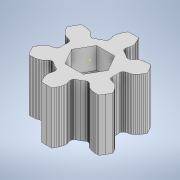
# Autodesk Inventor part: smallgears
Saved by Autodesk Inventor 2020 (Build 240168000, 168)
## iProperties
Created: 2019-08-05
Part Number: smallgears
Material: Generic
Document SubType Name: Modeling
Designer: erwin
Density: 1 g/cm^3
Appearance: Default
Author: erwin
Autodesk Inventor part; units mm, degrees
ref_plane "YZ Plane" through (0, 0, 0) normal (1, 0, 0) x (0, 1, 0)
ref_plane "XZ Plane" through (0, 0, 0) normal (0, 1, 0) x (-1, 0, 0)
ref_plane "XY Plane" through (0, 0, 0) normal (0, 0, 1) x (1, 0, 0)
sketch "Sketch1" plane through (0, 0, 0) normal (0, 1, 0) x (-1, 0, 0)
  line L0 (-11.846, 1.6672) -> (-11.8965, 2.1804)
  line L1 (-11.8965, 2.1804) -> (-11.9911, 2.3941)
  line L2 (-11.9911, 2.3941) -> (-12.094, 2.5558)
  line L3 (-12.094, 2.5558) -> (-12.2017, 2.6894)
  line L4 (-12.2017, 2.6894) -> (-12.3128, 2.8042)
  line L5 (-12.3128, 2.8042) -> (-12.4267, 2.905)
  line L6 (-12.4267, 2.905) -> (-12.6608, 3.0756)
  line L7 (-12.6608, 3.0756) -> (-12.902, 3.2145)
  line L8 (-12.902, 3.2145) -> (-13.1492, 3.3288)
  line L9 (-13.1492, 3.3288) -> (-13.6584, 3.4985)
  line L10 (-13.6584, 3.4985) -> (-14.1841, 3.6039)
  line L11 (-14.1841, 3.6039) -> (-14.7177, 3.6783)
  line L12 (-14.7177, 3.6783) -> (-15.2047, 3.9342)
  line L13 (-15.2047, 3.9342) -> (-15.6715, 4.2604)
  line L14 (-15.6715, 4.2604) -> (-16.1201, 4.6417)
  line L15 (-16.1201, 4.6417) -> (-16.5502, 5.0711)
  line L16 (-16.5502, 5.0711) -> (-16.961, 5.5447)
  line L17 (-16.961, 5.5447) -> (-17.3511, 6.0596)
  line L18 (-17.3511, 6.0596) -> (-17.7193, 6.6135)
  line L19 (-17.7193, 6.6135) -> (-18.064, 7.2045)
  line L20 (-18.064, 7.2045) -> (-18.3837, 7.831)
  line L21 (-18.3837, 7.831) -> (-17.3212, 9.9528)
  line L22 (-17.3212, 9.9528) -> (-16.0149, 11.9338)
  line L23 (-16.0149, 11.9338) -> (-15.3126, 11.9701)
  line L24 (-15.3126, 11.9701) -> (-14.6284, 11.9671)
  line L25 (-14.6284, 11.9671) -> (-13.9646, 11.9252)
  line L26 (-13.9646, 11.9252) -> (-13.3236, 11.8448)
  line L27 (-13.3236, 11.8448) -> (-12.7081, 11.7259)
  line L28 (-12.7081, 11.7259) -> (-12.1211, 11.5681)
  line L29 (-12.1211, 11.5681) -> (-11.5667, 11.3702)
  line L30 (-11.5667, 11.3702) -> (-11.0507, 11.1291)
  line L31 (-11.0507, 11.1291) -> (-10.5856, 10.8353)
  line L32 (-10.5856, 10.8353) -> (-10.2544, 10.4104)
  line L33 (-10.2544, 10.4104) -> (-9.9002, 10.0077)
  line L34 (-9.9002, 10.0077) -> (-9.4987, 9.6517)
  line L35 (-9.4987, 9.6517) -> (-9.2761, 9.4948)
  line L36 (-9.2761, 9.4948) -> (-9.0352, 9.3553)
  line L37 (-9.0352, 9.3553) -> (-8.7704, 9.2378)
  line L38 (-8.7704, 9.2378) -> (-8.6261, 9.1897)
  line L39 (-8.6261, 9.1897) -> (-8.4712, 9.1509)
  line L40 (-8.4712, 9.1509) -> (-8.3017, 9.1244)
  line L41 (-8.3017, 9.1244) -> (-8.1102, 9.1161)
  line L42 (-8.1102, 9.1161) -> (-7.8778, 9.141)
  line L43 (-7.8778, 9.141) -> (-7.4081, 9.3539)
  line L44 (-7.4081, 9.3539) -> (-5.9851, 10.318)
  line L45 (-5.9851, 10.318) -> (-4.4386, 11.0683)
  line L46 (-4.4386, 11.0683) -> (-4.0194, 11.3686)
  line L47 (-4.0194, 11.3686) -> (-3.8816, 11.5575)
  line L48 (-3.8816, 11.5575) -> (-3.7931, 11.7274)
  line L49 (-3.7931, 11.7274) -> (-3.7313, 11.8875)
  line L50 (-3.7313, 11.8875) -> (-3.6874, 12.0411)
  line L51 (-3.6874, 12.0411) -> (-3.657, 12.1901)
  line L52 (-3.657, 12.1901) -> (-3.6263, 12.4781)
  line L53 (-3.6263, 12.4781) -> (-3.6266, 12.7565)
  line L54 (-3.6266, 12.7565) -> (-3.6512, 13.0277)
  line L55 (-3.6512, 13.0277) -> (-3.7588, 13.5535)
  line L56 (-3.7588, 13.5535) -> (-3.9304, 14.0615)
  line L57 (-3.9304, 14.0615) -> (-4.1328, 14.5608)
  line L58 (-4.1328, 14.5608) -> (-4.1547, 15.1105)
  line L59 (-4.1547, 15.1105) -> (-4.1055, 15.6779)
  line L60 (-4.1055, 15.6779) -> (-3.9997, 16.257)
  line L61 (-3.9997, 16.257) -> (-3.8428, 16.8442)
  line L62 (-3.8428, 16.8442) -> (-3.6381, 17.4367)
  line L63 (-3.6381, 17.4367) -> (-3.3872, 18.0321)
  line L64 (-3.3872, 18.0321) -> (-3.0916, 18.6279)
  line L65 (-3.0916, 18.6279) -> (-2.7521, 19.2219)
  line L66 (-2.7521, 19.2219) -> (-2.3695, 19.812)
  line L67 (-2.3695, 19.812) -> (-0.0007, 19.9528)
  line L68 (-0.0007, 19.9528) -> (2.3681, 19.812)
  line L69 (2.3681, 19.812) -> (2.7507, 19.2219)
  line L70 (2.7507, 19.2219) -> (3.0902, 18.6279)
  line L71 (3.0902, 18.6279) -> (3.3858, 18.0321)
  line L72 (3.3858, 18.0321) -> (3.6366, 17.4367)
  line L73 (3.6366, 17.4367) -> (3.8414, 16.8442)
  line L74 (3.8414, 16.8442) -> (3.9983, 16.257)
  line L75 (3.9983, 16.257) -> (4.1041, 15.6779)
  line L76 (4.1041, 15.6779) -> (4.1533, 15.1105)
  line L77 (4.1533, 15.1105) -> (4.1314, 14.5608)
  line L78 (4.1314, 14.5608) -> (3.929, 14.0615)
  line L79 (3.929, 14.0615) -> (3.7574, 13.5535)
  line L80 (3.7574, 13.5535) -> (3.6498, 13.0277)
  line L81 (3.6498, 13.0277) -> (3.6252, 12.7565)
  line L82 (3.6252, 12.7565) -> (3.6249, 12.4781)
  line L83 (3.6249, 12.4781) -> (3.6555, 12.1901)
  line L84 (3.6555, 12.1901) -> (3.686, 12.0411)
  line L85 (3.686, 12.0411) -> (3.7298, 11.8875)
  line L86 (3.7298, 11.8875) -> (3.7917, 11.7274)
  line L87 (3.7917, 11.7274) -> (3.8802, 11.5575)
  line L88 (3.8802, 11.5575) -> (4.018, 11.3686)
  line L89 (4.018, 11.3686) -> (4.4372, 11.0683)
  line L90 (4.4372, 11.0683) -> (5.9837, 10.318)
  line L91 (5.9837, 10.318) -> (7.4067, 9.3539)
  line L92 (7.4067, 9.3539) -> (7.8764, 9.141)
  line L93 (7.8764, 9.141) -> (8.1088, 9.1161)
  line L94 (8.1088, 9.1161) -> (8.3002, 9.1244)
  line L95 (8.3002, 9.1244) -> (8.4698, 9.1509)
  line L96 (8.4698, 9.1509) -> (8.6247, 9.1897)
  line L97 (8.6247, 9.1897) -> (8.769, 9.2378)
  line L98 (8.769, 9.2378) -> (9.0338, 9.3553)
  line L99 (9.0338, 9.3553) -> (9.2747, 9.4948)
  line L100 (9.2747, 9.4948) -> (9.4972, 9.6517)
  line L101 (9.4972, 9.6517) -> (9.8988, 10.0077)
  line L102 (9.8988, 10.0077) -> (10.253, 10.4104)
  line L103 (10.253, 10.4104) -> (10.5842, 10.8353)
  line L104 (10.5842, 10.8353) -> (11.0493, 11.1291)
  line L105 (11.0493, 11.1291) -> (11.5653, 11.3702)
  line L106 (11.5653, 11.3702) -> (12.1197, 11.5681)
  line L107 (12.1197, 11.5681) -> (12.7067, 11.7259)
  line L108 (12.7067, 11.7259) -> (13.3222, 11.8448)
  line L109 (13.3222, 11.8448) -> (13.9632, 11.9252)
  line L110 (13.9632, 11.9252) -> (14.627, 11.9671)
  line L111 (14.627, 11.9671) -> (15.3112, 11.9701)
  line L112 (15.3112, 11.9701) -> (16.0135, 11.9338)
  line L113 (16.0135, 11.9338) -> (17.3198, 9.9528)
  line L114 (17.3198, 9.9528) -> (18.3823, 7.831)
  line L115 (18.3823, 7.831) -> (18.0626, 7.2045)
  line L116 (18.0626, 7.2045) -> (17.7179, 6.6135)
  line L117 (17.7179, 6.6135) -> (17.3497, 6.0596)
  line L118 (17.3497, 6.0596) -> (16.9595, 5.5447)
  line L119 (16.9595, 5.5447) -> (16.5488, 5.0711)
  line L120 (16.5488, 5.0711) -> (16.1187, 4.6417)
  line L121 (16.1187, 4.6417) -> (15.6701, 4.2604)
  line L122 (15.6701, 4.2604) -> (15.2033, 3.9342)
  line L123 (15.2033, 3.9342) -> (14.7163, 3.6783)
  line L124 (14.7163, 3.6783) -> (14.1827, 3.6039)
  line L125 (14.1827, 3.6039) -> (13.6569, 3.4985)
  line L126 (13.6569, 3.4985) -> (13.1478, 3.3288)
  line L127 (13.1478, 3.3288) -> (12.9006, 3.2145)
  line L128 (12.9006, 3.2145) -> (12.6594, 3.0756)
  line L129 (12.6594, 3.0756) -> (12.4253, 2.905)
  line L130 (12.4253, 2.905) -> (12.3114, 2.8042)
  line L131 (12.3114, 2.8042) -> (12.2003, 2.6894)
  line L132 (12.2003, 2.6894) -> (12.0926, 2.5558)
  line L133 (12.0926, 2.5558) -> (11.9897, 2.3941)
  line L134 (11.9897, 2.3941) -> (11.8951, 2.1804)
  line L135 (11.8951, 2.1804) -> (11.8446, 1.6672)
  line L136 (11.8446, 1.6672) -> (11.968, -0.0472)
  line L137 (11.968, -0.0472) -> (11.8446, -1.7617)
  line L138 (11.8446, -1.7617) -> (11.8951, -2.2749)
  line L139 (11.8951, -2.2749) -> (11.9897, -2.4886)
  line L140 (11.9897, -2.4886) -> (12.0926, -2.6503)
  line L141 (12.0926, -2.6503) -> (12.2003, -2.7838)
  line L142 (12.2003, -2.7838) -> (12.3114, -2.8986)
  line L143 (12.3114, -2.8986) -> (12.4253, -2.9995)
  line L144 (12.4253, -2.9995) -> (12.6594, -3.17)
  line L145 (12.6594, -3.17) -> (12.9006, -3.309)
  line L146 (12.9006, -3.309) -> (13.1478, -3.4232)
  line L147 (13.1478, -3.4232) -> (13.6569, -3.593)
  line L148 (13.6569, -3.593) -> (14.1827, -3.6984)
  line L149 (14.1827, -3.6984) -> (14.7163, -3.7728)
  line L150 (14.7163, -3.7728) -> (15.2033, -4.0286)
  line L151 (15.2033, -4.0286) -> (15.6701, -4.3549)
  line L152 (15.6701, -4.3549) -> (16.1187, -4.7361)
  line L153 (16.1187, -4.7361) -> (16.5488, -5.1656)
  line L154 (16.5488, -5.1656) -> (16.9595, -5.6392)
  line L155 (16.9595, -5.6392) -> (17.3497, -6.1541)
  line L156 (17.3497, -6.1541) -> (17.7179, -6.708)
  line L157 (17.7179, -6.708) -> (18.0626, -7.299)
  line L158 (18.0626, -7.299) -> (18.3823, -7.9254)
  line L159 (18.3823, -7.9254) -> (17.3198, -10.0472)
  line L160 (17.3198, -10.0472) -> (16.0135, -12.0283)
  line L161 (16.0135, -12.0283) -> (15.3112, -12.0646)
  line L162 (15.3112, -12.0646) -> (14.627, -12.0616)
  line L163 (14.627, -12.0616) -> (13.9632, -12.0197)
  line L164 (13.9632, -12.0197) -> (13.3222, -11.9393)
  line L165 (13.3222, -11.9393) -> (12.7067, -11.8204)
  line L166 (12.7067, -11.8204) -> (12.1197, -11.6626)
  line L167 (12.1197, -11.6626) -> (11.5653, -11.4647)
  line L168 (11.5653, -11.4647) -> (11.0493, -11.2236)
  line L169 (11.0493, -11.2236) -> (10.5842, -10.9298)
  line L170 (10.5842, -10.9298) -> (10.253, -10.5049)
  line L171 (10.253, -10.5049) -> (9.8988, -10.1022)
  line L172 (9.8988, -10.1022) -> (9.4972, -9.7462)
  line L173 (9.4972, -9.7462) -> (9.2747, -9.5893)
  line L174 (9.2747, -9.5893) -> (9.0338, -9.4498)
  line L175 (9.0338, -9.4498) -> (8.769, -9.3323)
  line L176 (8.769, -9.3323) -> (8.6247, -9.2842)
  line L177 (8.6247, -9.2842) -> (8.4698, -9.2453)
  line L178 (8.4698, -9.2453) -> (8.3002, -9.2188)
  line L179 (8.3002, -9.2188) -> (8.1088, -9.2106)
  line L180 (8.1088, -9.2106) -> (7.8764, -9.2355)
  line L181 (7.8764, -9.2355) -> (7.4067, -9.4484)
  line L182 (7.4067, -9.4484) -> (5.9837, -10.4125)
  line L183 (5.9837, -10.4125) -> (4.4372, -11.1628)
  line L184 (4.4372, -11.1628) -> (4.018, -11.4631)
  line L185 (4.018, -11.4631) -> (3.8802, -11.6519)
  line L186 (3.8802, -11.6519) -> (3.7917, -11.8219)
  line L187 (3.7917, -11.8219) -> (3.7298, -11.9819)
  line L188 (3.7298, -11.9819) -> (3.686, -12.1356)
  line L189 (3.686, -12.1356) -> (3.6555, -12.2846)
  line L190 (3.6555, -12.2846) -> (3.6249, -12.5726)
  line L191 (3.6249, -12.5726) -> (3.6252, -12.851)
  line L192 (3.6252, -12.851) -> (3.6498, -13.1222)
  line L193 (3.6498, -13.1222) -> (3.7574, -13.648)
  line L194 (3.7574, -13.648) -> (3.929, -14.156)
  line L195 (3.929, -14.156) -> (4.1314, -14.6553)
  line L196 (4.1314, -14.6553) -> (4.1533, -15.205)
  line L197 (4.1533, -15.205) -> (4.1041, -15.7724)
  line L198 (4.1041, -15.7724) -> (3.9983, -16.3515)
  line L199 (3.9983, -16.3515) -> (3.8414, -16.9387)
  line L200 (3.8414, -16.9387) -> (3.6366, -17.5312)
  line L201 (3.6366, -17.5312) -> (3.3858, -18.1266)
  line L202 (3.3858, -18.1266) -> (3.0902, -18.7223)
  line L203 (3.0902, -18.7223) -> (2.7507, -19.3164)
  line L204 (2.7507, -19.3164) -> (2.3681, -19.9065)
  line L205 (2.3681, -19.9065) -> (-0.0007, -20.0472)
  line L206 (-0.0007, -20.0472) -> (-2.3695, -19.9065)
  line L207 (-2.3695, -19.9065) -> (-2.7521, -19.3164)
  line L208 (-2.7521, -19.3164) -> (-3.0916, -18.7223)
  line L209 (-3.0916, -18.7223) -> (-3.3872, -18.1266)
  line L210 (-3.3872, -18.1266) -> (-3.6381, -17.5312)
  line L211 (-3.6381, -17.5312) -> (-3.8428, -16.9387)
  line L212 (-3.8428, -16.9387) -> (-3.9997, -16.3515)
  line L213 (-3.9997, -16.3515) -> (-4.1055, -15.7724)
  line L214 (-4.1055, -15.7724) -> (-4.1547, -15.205)
  line L215 (-4.1547, -15.205) -> (-4.1328, -14.6553)
  line L216 (-4.1328, -14.6553) -> (-3.9304, -14.156)
  line L217 (-3.9304, -14.156) -> (-3.7588, -13.648)
  line L218 (-3.7588, -13.648) -> (-3.6512, -13.1222)
  line L219 (-3.6512, -13.1222) -> (-3.6266, -12.851)
  line L220 (-3.6266, -12.851) -> (-3.6263, -12.5726)
  line L221 (-3.6263, -12.5726) -> (-3.657, -12.2846)
  line L222 (-3.657, -12.2846) -> (-3.6874, -12.1356)
  line L223 (-3.6874, -12.1356) -> (-3.7313, -11.9819)
  line L224 (-3.7313, -11.9819) -> (-3.7931, -11.8219)
  line L225 (-3.7931, -11.8219) -> (-3.8816, -11.6519)
  line L226 (-3.8816, -11.6519) -> (-4.0194, -11.4631)
  line L227 (-4.0194, -11.4631) -> (-4.4386, -11.1628)
  line L228 (-4.4386, -11.1628) -> (-5.9851, -10.4125)
  line L229 (-5.9851, -10.4125) -> (-7.4081, -9.4484)
  line L230 (-7.4081, -9.4484) -> (-7.8778, -9.2355)
  line L231 (-7.8778, -9.2355) -> (-8.1102, -9.2106)
  line L232 (-8.1102, -9.2106) -> (-8.3017, -9.2188)
  line L233 (-8.3017, -9.2188) -> (-8.4712, -9.2453)
  line L234 (-8.4712, -9.2453) -> (-8.6261, -9.2842)
  line L235 (-8.6261, -9.2842) -> (-8.7704, -9.3323)
  line L236 (-8.7704, -9.3323) -> (-9.0352, -9.4498)
  line L237 (-9.0352, -9.4498) -> (-9.2761, -9.5893)
  line L238 (-9.2761, -9.5893) -> (-9.4987, -9.7462)
  line L239 (-9.4987, -9.7462) -> (-9.9002, -10.1022)
  line L240 (-9.9002, -10.1022) -> (-10.2544, -10.5049)
  line L241 (-10.2544, -10.5049) -> (-10.5856, -10.9298)
  line L242 (-10.5856, -10.9298) -> (-11.0507, -11.2236)
  line L243 (-11.0507, -11.2236) -> (-11.5667, -11.4647)
  line L244 (-11.5667, -11.4647) -> (-12.1211, -11.6626)
  line L245 (-12.1211, -11.6626) -> (-12.7081, -11.8204)
  line L246 (-12.7081, -11.8204) -> (-13.3236, -11.9393)
  line L247 (-13.3236, -11.9393) -> (-13.9646, -12.0197)
  line L248 (-13.9646, -12.0197) -> (-14.6284, -12.0616)
  line L249 (-14.6284, -12.0616) -> (-15.3126, -12.0646)
  line L250 (-15.3126, -12.0646) -> (-16.0149, -12.0283)
  line L251 (-16.0149, -12.0283) -> (-17.3212, -10.0472)
  line L252 (-17.3212, -10.0472) -> (-18.3837, -7.9254)
  line L253 (-18.3837, -7.9254) -> (-18.064, -7.299)
  line L254 (-18.064, -7.299) -> (-17.7193, -6.708)
  line L255 (-17.7193, -6.708) -> (-17.3511, -6.1541)
  line L256 (-17.3511, -6.1541) -> (-16.961, -5.6392)
  line L257 (-16.961, -5.6392) -> (-16.5502, -5.1656)
  line L258 (-16.5502, -5.1656) -> (-16.1201, -4.7361)
  line L259 (-16.1201, -4.7361) -> (-15.6715, -4.3549)
  line L260 (-15.6715, -4.3549) -> (-15.2047, -4.0286)
  line L261 (-15.2047, -4.0286) -> (-14.7177, -3.7728)
  line L262 (-14.7177, -3.7728) -> (-14.1841, -3.6984)
  line L263 (-14.1841, -3.6984) -> (-13.6584, -3.593)
  line L264 (-13.6584, -3.593) -> (-13.1492, -3.4232)
  line L265 (-13.1492, -3.4232) -> (-12.902, -3.309)
  line L266 (-12.902, -3.309) -> (-12.6608, -3.17)
  line L267 (-12.6608, -3.17) -> (-12.4267, -2.9995)
  line L268 (-12.4267, -2.9995) -> (-12.3128, -2.8986)
  line L269 (-12.3128, -2.8986) -> (-12.2017, -2.7838)
  line L270 (-12.2017, -2.7838) -> (-12.094, -2.6503)
  line L271 (-12.094, -2.6503) -> (-11.9911, -2.4886)
  line L272 (-11.9911, -2.4886) -> (-11.8965, -2.2749)
  line L273 (-11.8965, -2.2749) -> (-11.846, -1.7617)
  line L274 (-11.846, -1.7617) -> (-11.9694, -0.0472)
  line L275 (-11.9694, -0.0472) -> (-11.846, 1.6672)
  circle A0 centre (0, 0) radius 4.75
  point P0 (0, 0)
  point P1 (3.9983, 16.257)
  point P2 (-0.0007, 19.9528)
  point P3 (4.018, -11.4631)
  point P4 (4.4372, -11.1628)
  dimension "d0" = 40
  dimension "d4" = 10.318
  dimension "d5" = 5.9837
  constraints: 552 end point, 1 centre point
  measures "d0" distance of L205.end L67.end
  measures "d4" vertical distance of L90.end A0.centre
  measures "d5" horizontal distance of L90.end A0.centre
extrude "Extrusion1" add sketch "Sketch1" along normal blind 24
sketch "Sketch2" plane through (0, 24, 0) normal (0, 1, 0) x (1, 0, 0)
  point P0 (0, 0)
sketch "Sketch3" plane through (0, 24, 0) normal (0, 1, 0) x (1, 0, 0)
  line L0 (-8.3716, 0) -> (-4.1858, 7.25)
  line L1 (-4.1858, 7.25) -> (4.1858, 7.25)
  line L2 (4.1858, 7.25) -> (8.3716, 0)
  line L3 (8.3716, 0) -> (4.1858, -7.25)
  line L4 (4.1858, -7.25) -> (-4.1858, -7.25)
  line L5 (-4.1858, -7.25) -> (-8.3716, 0)
  point P0 (0, 0)
  point P1 (0, 0)
  dimension "d6" = 14.5
  constraints: 12 end point, 1 coincident, 13 other
  measures "d6" distance between parallel lines of L3 L0
extrude "Extrusion2" cut sketch "Sketch3" against normal blind 10
sketch "Sketch4" plane through (0, 0, 0) normal (0, -1, 0) x (1, 0, 0)
  circle A0 centre (0, 0) radius 8
  dimension "d9" = 16
  constraints: 1 centre point, 1 coincident
  measures "d9" diameter of A0
extrude "Extrusion3" cut sketch "Sketch4" against normal blind 5
body "Solid1"
